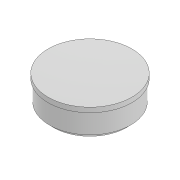
# Autodesk Inventor part: Dust Filter
Saved by Autodesk Inventor 2020 (Build 240168000, 168)
## iProperties
Created: 2020-04-08
Part Number: Dust Filter
Material: Generic
Document SubType Name: Modeling
Designer: angusaitken
Density: 1 g/cm^3
Appearance: Default
Description: N95 CANISTER FILTER
Author: angusaitken
Autodesk Inventor part; units mm, degrees
ref_plane "YZ Plane" through (0, 0, 0) normal (1, 0, 0) x (0, 1, 0)
ref_plane "XZ Plane" through (0, 0, 0) normal (0, 1, 0) x (-1, 0, 0)
ref_plane "XY Plane" through (0, 0, 0) normal (0, 0, 1) x (1, 0, 0)
sketch "Sketch1" plane through (0, 0, 0) normal (0, 1, 0) x (-1, 0, 0)
  circle A0 centre (0, 0) radius 19
  dimension "d0" = 38
  constraints: 1 centre point, 1 coincident
  measures "d0" diameter of A0
extrude "Extrusion1" add sketch "Sketch1" along normal blind 5.4
sketch "Sketch2" plane through (0, 5.4, 0) normal (0, 1, 0) x (1, 0, 0)
  circle A0 centre (0, 0) radius 38.125
  dimension "d3" = 76.25
  constraints: 1 centre point, 1 coincident
  measures "d3" diameter of A0
extrude "Extrusion2" add sketch "Sketch2" along normal blind 4.35
sketch "Sketch3" plane through (0, 9.75, 0) normal (0, 1, 0) x (1, 0, 0)
  circle A0 centre (0, 0) radius 42.4
  dimension "d6" = 84.8
  constraints: 1 centre point, 1 coincident
  measures "d6" diameter of A0
extrude "Extrusion3" add sketch "Sketch3" along normal blind 21
sketch "Sketch4" plane through (0, 30.75, 0) normal (0, 1, 0) x (1, 0, 0)
  circle A0 centre (0, 0) radius 43.8
  dimension "d9" = 87.6
  constraints: 1 centre point, 1 coincident
  measures "d9" diameter of A0
extrude "Extrusion4" add sketch "Sketch4" along normal blind 5
sketch "Sketch5" plane through (0, 0, 0) normal (1, 0, 0) x (0, 1, 0)
  line L0 (35.75, -43.8) -> (35.75, 43.8) projected
  line L1 (35.75, -43.8) -> (35.75, 43.8) projected
  line L2 (30.75, -43.8) -> (30.75, 43.8)
  line L3 (35.75, 0) -> (40.75, 0)
  arc A0 (40.75, 0) -> (35.75, 43.8) centre (-179.7193, -2.9823) ccw
  line L4 (35.75, 0) -> (35.75, 43.8)
  point P0 (0, 0)
  dimension "d12" = 5
  constraints: 6 end point, 2 point on circle, 1 centre point, 1 horizontal
  measures "d12" distance of L3.start L3.end
revolve "Revolution1" add sketch "Sketch5" angle 360 about axis through (0, 35.75, 0) along (0, 1, 0)
body "Solid1"
